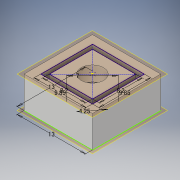
# Autodesk Inventor part: pin_joint_plastic_ver2
Saved by Autodesk Inventor 2019 (Build 230136000, 136)
## iProperties
Created: 2019-08-27
Part Number: pin_joint_plastic_ver2
Material: Generic
Document SubType Name: Modeling
Designer: ushiyama
Density: 1 g/cm^3
Appearance: Default
Author: ushiyama
Autodesk Inventor part; units mm, degrees
ref_plane "YZ Plane" through (0, 0, 0) normal (1, 0, 0) x (0, 1, 0)
ref_plane "XY Plane" through (0, 0, 0) normal (0, 0, 1) x (1, 0, 0)
ref_plane "作業平面2" through (0, 6, 0) normal (0, 1, 0) x (-1, 0, 0)
sketch "スケッチ3" plane through (0, 6, 0) normal (0, 1, 0) x (-1, 0, 0)
  line L0 (4.1, -4.1) -> (-4.1, -4.1)
  line L1 (-4.1, -4.1) -> (-4.1, 4.1)
  line L2 (-4.1, 4.1) -> (4.1, 4.1)
  line L3 (4.1, 4.1) -> (4.1, -4.1)
  line L4 (4.1, -4.1) -> (-4.1, 4.1) construction
  line L5 (-4.1, -4.1) -> (4.1, 4.1) construction
  line L6 (4.925, -4.925) -> (-4.925, -4.925)
  line L7 (-4.925, -4.925) -> (-4.925, 4.925)
  line L8 (-4.925, 4.925) -> (4.925, 4.925)
  line L9 (4.925, 4.925) -> (4.925, -4.925)
  line L10 (4.925, -4.925) -> (-4.925, 4.925) construction
  line L11 (-4.925, -4.925) -> (4.925, 4.925) construction
  point P0 (0, 0)
  point P1 (0, 0)
  dimension "d19" = 8.2
  dimension "d20" = 8.2
  dimension "d21" = 9.85
  dimension "d22" = 9.85
  constraints: 24 end point, 4 midpoint, 4 parallel, 2 horizontal, 2 perpendicular, 1 coincident
  measures "d19" distance of L1.end L2.end
  measures "d20" distance of L0.end L1.end
  measures "d21" distance of L7.end L8.end
  measures "d22" distance of L6.end L7.end
sketch "スケッチ1" plane through (0, 0, 0) normal (0, 1, 0) x (-1, 0, 0)
  line L0 (6.5, -6.5) -> (-6.5, 6.5) construction
  line L1 (-6.5, -6.5) -> (6.5, 6.5) construction
  line L2 (1.046, 3.9037) -> (3.9037, 1.046)
  line L3 (3.9037, 1.046) -> (2.8577, -2.8577)
  line L4 (2.8577, -2.8577) -> (-1.046, -3.9037)
  line L5 (-1.046, -3.9037) -> (-3.9037, -1.046)
  line L6 (-3.9037, -1.046) -> (-2.8577, 2.8577)
  line L7 (-2.8577, 2.8577) -> (1.046, 3.9037)
  line L8 (-6.5, -6.5) -> (6.5, -6.5)
  line L9 (6.5, -6.5) -> (6.5, 6.5)
  line L10 (6.5, 6.5) -> (-6.5, 6.5)
  line L11 (-6.5, 6.5) -> (-6.5, -6.5)
  line L12 (-6.5, -6.5) -> (6.5, 6.5) construction
  line L13 (6.5, -6.5) -> (-6.5, 6.5) construction
  circle A0 centre (0, 0) radius 2.125
  dimension "d33" = 7
  dimension "d34" = 13
  dimension "d35" = 13
  dimension "d36" = 4.25
  constraints: 28 end point, 3 midpoint, 3 parallel, 1 centre point, 1 coincident, 1 horizontal, 1 perpendicular, 13 other
  measures "d33" distance between parallel lines of L2 L5
  measures "d34" distance of L10.end L1.end
  measures "d35" distance of L1.end L8.end
  measures "d36" diameter of A0
extrude "押し出し8" add sketch "スケッチ1" along normal blind 6 contours L2 L3 L4 L5 L6 L7 | L11 L10 L9 L8 | A0
extrude "押し出し9" cut sketch "スケッチ3" against normal blind 2
extrude "押し出し10" cut sketch "スケッチ1" along normal blind 3.2 contours L2 L3 L4 L5 L6 L7
extrude "押し出し11" cut sketch "スケッチ1" along normal blind 6 contours A0
